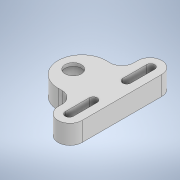
# Autodesk Inventor part: Lampenhalterung1,0
Saved by Autodesk Inventor 2021.3 (Build 253353000, 353)
## iProperties
Created: 2021-10-11
Part Number: Lampenhalterung1,0
Material: Generisch
Document SubType Name: Modeling
Designer: bhelg
Density: 1 g/cm^3
Appearance: Vorgabe
Author: bhelg
Autodesk Inventor part; units mm, degrees
ref_plane "YZ Plane" through (0, 0, 0) normal (1, 0, 0) x (0, 1, 0)
ref_plane "XZ Plane" through (0, 0, 0) normal (0, 1, 0) x (-1, 0, 0)
ref_plane "XY Plane" through (0, 0, 0) normal (0, 0, 1) x (1, 0, 0)
sketch "Skizze1" plane through (0, 0, 0) normal (0, 1, 0) x (-1, 0, 0)
  line L0 (0, 0) -> (15, 0)
  line L1 (15, 0) -> (15, -17.5)
  line L2 (15, -17.5) -> (40, -17.5)
  line L3 (40, -17.5) -> (40, -47.5)
  line L4 (40, -47.5) -> (15, -47.5)
  line L5 (15, -47.5) -> (15, -65)
  line L6 (15, -65) -> (0, -65)
  line L7 (0, -65) -> (0, 0)
  dimension "d0" = 65
  dimension "d1" = 30
  dimension "d2" = 15
  dimension "d3" = 40
  dimension "d6" = 25
  constraints: 16 end point, 6 perpendicular, 2 point on line, 1 collinear, 1 horizontal
  measures "d0" distance of L6.end L0.start
  measures "d1" distance between parallel lines of L4 L2
  measures "d2" distance between parallel lines of L1 L7
  measures "d3" distance between parallel lines of L3 L7
  measures "d6" distance between parallel lines of L3 L5
extrude "Extrusion3" add sketch "Skizze1" along normal blind 12
sketch "Skizze5" plane through (0, 0, 0) normal (0, -1, 0) x (1, 0, 0)
  line L0 (-7.5, -58) -> (-7.5, -43) construction
  line L1 (-4.95, -58) -> (-4.95, -43)
  line L2 (-10.05, -43) -> (-10.05, -58)
  arc A0 (-10.05, -58) -> (-4.95, -58) centre (-7.5, -58) ccw
  arc A1 (-4.95, -43) -> (-10.05, -43) centre (-7.5, -43) ccw
  line L3 (-7.5, -22) -> (-7.5, -7) construction
  line L4 (-4.95, -22) -> (-4.95, -7)
  line L5 (-10.05, -7) -> (-10.05, -22)
  arc A2 (-10.05, -22) -> (-4.95, -22) centre (-7.5, -22) ccw
  arc A3 (-4.95, -7) -> (-10.05, -7) centre (-7.5, -7) ccw
  line L6 (0, -65) -> (-15, -65) projected
  line L7 (-15, 0) -> (0, 0) projected
  line L8 (-15, -65) -> (-15, -47.5) projected
  line L9 (0, 0) -> (0, -65) projected
  point P0 (-7.5, -50.5)
  point P1 (-7.5, -14.5)
  dimension "d52" = 5.1
  dimension "d53" = 5.1
  dimension "d54" = 15
  dimension "d55" = 15
  dimension "d56" = 7
  dimension "d58" = 7
  dimension "d59" = 15
  dimension "d60" = 7.5
  dimension "d76" = 36
  constraints: 16 end point, 8 point on circle, 8 tangent, 4 centre point, 2 midpoint, 2 parallel, 2 point on line, 1 vertical
  measures "d52" distance between parallel lines of L1 L2
  measures "d53" distance between parallel lines of L4 L5
  measures "d54" distance of L0.end L0.start
  measures "d55" distance of L3.end L3.start
  measures "d56" distance from line of L6 L0.start
  measures "d58" distance from line of L3.end L7
  measures "d59" distance between parallel lines of L8 L9
  measures "d60" distance between parallel lines of L0 L9
  measures "d76" distance of point (-7.5, -14.5) point (-7.5, -50.5)
extrude "Extrusion5" cut sketch "Skizze5" against normal through all
sketch "Skizze6" plane through (0, 0, 0) normal (0, -1, 0) x (1, 0, 0)
  line L0 (-7.5, -58) -> (-7.5, -43) construction
  line L1 (-2.5, -58) -> (-2.5, -43)
  line L2 (-12.5, -43) -> (-12.5, -58)
  arc A0 (-12.5, -58) -> (-2.5, -58) centre (-7.5, -58) ccw
  arc A1 (-2.5, -43) -> (-12.5, -43) centre (-7.5, -43) ccw
  line L3 (-7.5, -22) -> (-7.5, -7) construction
  line L4 (-2.5, -22) -> (-2.5, -7)
  line L5 (-12.5, -7) -> (-12.5, -22)
  arc A2 (-12.5, -22) -> (-2.5, -22) centre (-7.5, -22) ccw
  arc A3 (-2.5, -7) -> (-12.5, -7) centre (-7.5, -7) ccw
  line L6 (-15, 0) -> (0, 0) projected
  line L7 (0, 0) -> (0, -65) projected
  point P0 (-7.5, -50.5)
  point P1 (-7.5, -14.5)
  dimension "d63" = 10
  dimension "d64" = 10
  dimension "d65" = 15
  dimension "d66" = 15
  dimension "d67" = 7
  dimension "d68" = 7.5
  dimension "d69" = 7.5
  dimension "d70" = 7
  constraints: 16 end point, 8 point on circle, 8 tangent, 4 centre point, 3 parallel, 2 midpoint, 1 vertical
  measures "d63" distance between parallel lines of L2 L1
  measures "d64" distance between parallel lines of L4 L5
  measures "d65" distance of L0.end L0.start
  measures "d66" distance of L3.end L3.start
  measures "d67" distance from line of L6 L3.end
  measures "d68" distance from line of L3.end L7
  measures "d69" distance from line of L0.start L7
  measures "d70" vertical distance of L7.end L0.start
extrude "Extrusion6" cut sketch "Skizze6" against normal blind 5
fillet "Rundung4" radius 7.5 6 edges at (-15, 6, -65) (0, 6, -65) (0, 6, 0) (-15, 6, 0) (-15, 6, -17.5) (-15, 6, -47.5)
fillet "Rundung5" radius 15 2 edges at (-40, 6, -47.5) (-40, 6, -17.5)
sketch "Skizze7" plane through (0, 0, 0) normal (0, -1, 0) x (1, 0, 0)
  circle A0 centre (-30.5, -32.5) radius 3.7991
  point P0 (0, 0)
  dimension "d77" = 32.5
  dimension "d78" = 30.5
  constraints: 1 centre point
  measures "d77" vertical distance of A0.centre point (0, 0)
  measures "d78" horizontal distance of point (0, 0) A0.centre
hole "Bohrung1" at (-30.5, 0, -32.5) direction (0, 1, 0) diameter 10.2 end through all counterbore diameter 17 counterbore depth 10
